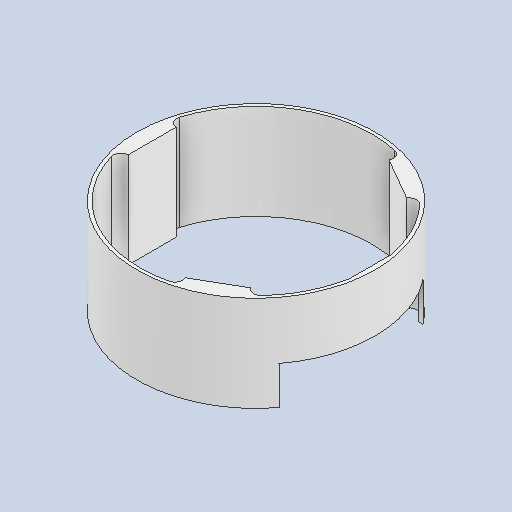
# Autodesk Inventor part: allwall
Saved by Autodesk Inventor 2023 (Build 270158000, 158)
## iProperties
Created: 2022-12-04
Part Number: allwall
Material: PC/ABS プラスチック
Document SubType Name: Modeling
Designer: RiSA
Density: 0.357273 g/cm^3
Appearance: 滑らか - 白
Author: RiSA
Autodesk Inventor part; units mm, degrees
ref_plane "YZ Plane" through (0, 0, 0) normal (1, 0, 0) x (0, 1, 0)
ref_plane "XZ Plane" through (0, 0, 0) normal (0, 1, 0) x (-1, 0, 0)
ref_plane "XY Plane" through (0, 0, 0) normal (0, 0, 1) x (1, 0, 0)
sketch "スケッチ1" plane through (0, 0, 0) normal (0, 1, 0) x (-1, 0, 0)
  circle A0 centre (0, 0) radius 125
  circle A1 centre (0, 0) radius 121.5
  line L0 (118.86, 0) -> (118.86, -25.1903)
  line L1 (118.86, 0) -> (118.86, 25.1903)
  line L2 (118.86, 25.1903) -> (108.86, 25.1903)
  line L3 (108.86, 25.1903) -> (108.86, -25.1903)
  line L4 (108.86, -25.1903) -> (118.86, -25.1903)
  line L5 (118.86, -25.1903) -> (118.86, 25.1903)
  line L6 (-59.43, 102.9358) -> (-37.6146, 115.5309)
  line L7 (-59.43, 102.9358) -> (-81.2454, 90.3406)
  line L8 (-81.2454, 90.3406) -> (-76.2454, 81.6804)
  line L9 (-76.2454, 81.6804) -> (-32.6146, 106.8707)
  line L10 (-32.6146, 106.8707) -> (-37.6146, 115.5309)
  line L11 (-37.6146, 115.5309) -> (-81.2454, 90.3406)
  line L12 (-59.43, -102.9358) -> (-81.2454, -90.3406)
  line L13 (-59.43, -102.9358) -> (-37.6146, -115.5309)
  line L14 (-37.6146, -115.5309) -> (-32.6146, -106.8707)
  line L15 (-32.6146, -106.8707) -> (-76.2454, -81.6804)
  line L16 (-76.2454, -81.6804) -> (-81.2454, -90.3406)
  line L17 (-81.2454, -90.3406) -> (-37.6146, -115.5309)
  dimension "d0" = 250
  dimension "d1" = 243
  dimension "d2" = 118.86
  dimension "d3" = 10
  dimension "d6" = 360
  constraints: 36 end point, 3 point on line, 2 centre point, 2 coincident, 2 parallel, 2 point on circle, 1 horizontal, 1 perpendicular, 1 vertical, 37 other
  measures "d0" diameter of A0
  measures "d1" diameter of A1
  measures "d2" distance of A1.centre L0.start
  measures "d3" distance of L4.end L3.end
extrude "押し出し1" add sketch "スケッチ1" along normal blind 100 contours A0 | A1 L0 L1 | L1 L0 L4 L3 L2 | L6 L7 A1 | L10 L9 L8 L7 L6 | A1 L12 L13 | L13 L12 L16 L15 L14
fillet "フィレット1" radius 8 6 edges at (37.6146, 50, -115.5309) (81.2454, 50, -90.3406) (-118.86, 50, 25.1903) (-118.86, 50, -25.1903) (81.2454, 50, 90.3406) (37.6146, 50, 115.5309)
sketch "スケッチ4" plane through (0, 100, 0) normal (0, 1, 0) x (1, 0, 0)
  line L0 (119.6242, 0) -> (119.6242, -21.2671)
  arc A0 (88.8593, -82.863) -> (88.8593, 82.863) centre (0, 0) ccw projected
  line L1 (119.6242, 0) -> (119.6242, 21.2671)
  arc A1 (119.6242, -21.2671) -> (119.6242, 21.2671) centre (0, 0) ccw
  constraints: 4 end point, 4 point on circle, 1 centre point, 1 point on line, 1 vertical
extrude "押し出し4" add sketch "スケッチ4" against normal blind 100
sketch "スケッチ5" plane through (119.6242, 100, -21.2671) normal (-1, 0, 0) x (0, 0, 1)
  line L0 (96.7671, -100) -> (-54.2329, -100)
  line L1 (-54.2329, -100) -> (-54.2329, -64.5)
  line L2 (-54.2329, -64.5) -> (96.7671, -64.5)
  line L3 (96.7671, -64.5) -> (96.7671, -100)
  line L4 (96.7671, -100) -> (-54.2329, -64.5) construction
  line L5 (-54.2329, -100) -> (96.7671, -64.5) construction
  line L6 (42.5342, -100) -> (0, -100) projected
  point P0 (21.2671, -100)
  point P1 (21.2671, -82.25)
  dimension "d20" = 151
  dimension "d21" = 35.5
  dimension "d22" = 0
  constraints: 12 end point, 2 midpoint, 2 parallel, 1 horizontal, 1 perpendicular
  measures "d20" distance of L1.end L2.end
  measures "d21" distance of L0.end L1.end
  measures "d22" distance between parallel lines of L6 L0
extrude "押し出し5" add sketch "スケッチ5" along normal blind 30
sketch "スケッチ6" plane through (89.6242, 100, -21.2671) normal (-1, 0, 0) x (0, 0, 1)
  line L0 (96.7671, -64.5) -> (-54.2329, -64.5) projected
  line L1 (-54.2329, -100) -> (96.7671, -100) projected
  line L2 (-54.2329, -64.5) -> (96.7671, -64.5)
  line L3 (96.7671, -64.5) -> (96.7671, -100)
  line L4 (96.7671, -100) -> (-54.2329, -100)
  line L5 (-54.2329, -100) -> (-54.2329, -64.5)
  line L6 (-54.2329, -64.5) -> (-54.2329, -100) projected
  line L7 (-54.2329, -64.5) -> (96.7671, -64.5)
  line L8 (96.7671, -64.5) -> (96.7671, -60)
  line L9 (96.7671, -60) -> (-54.2329, -60)
  line L10 (-54.2329, -60) -> (-54.2329, -64.5)
  point P0 (21.2671, -100)
  point P1 (-54.2329, -100)
  dimension "d27" = 151
  dimension "d28" = 4.5
  constraints: 16 end point, 4 parallel, 2 horizontal, 2 perpendicular
  measures "d27" distance of L9.end L8.end
  measures "d28" distance of L8.end L7.end
extrude "押し出し6" cut sketch "スケッチ6" against normal blind 100
